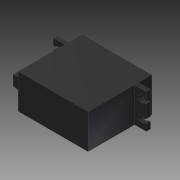
# Autodesk Inventor part: serwo HX12K
Saved by Autodesk Inventor 2013 (Build 170138000, 138)
## iProperties
Created: 2013-03-06
Part Number: serwo HX12K
Material: Generic
Document SubType Name: Modeling
Designer: Masta
Density: 1 g/cm^3
Author: Masta
Autodesk Inventor part; units mm, degrees
ref_plane "YZ Plane" through (0, 0, 0) normal (1, 0, 0) x (0, 1, 0)
ref_plane "XZ Plane" through (0, 0, 0) normal (0, 1, 0) x (-1, 0, 0)
ref_plane "XY Plane" through (0, 0, 0) normal (0, 0, 1) x (1, 0, 0)
sketch "Sketch1" plane through (0, 0, 0) normal (0, 1, 0) x (-1, 0, 0)
  line L0 (20.25, 10) -> (-20.25, 10)
  line L1 (-20.25, 10) -> (-20.25, -10)
  line L2 (-20.25, -10) -> (20.25, -10)
  line L3 (20.25, -10) -> (20.25, 10)
  line L4 (20.25, 10) -> (-20.25, -10) construction
  line L5 (-20.25, 10) -> (20.25, -10) construction
  line L6 (-27, 10) -> (-27, 6.25)
  line L7 (27, -10) -> (27, -6.25)
  line L8 (27, 10) -> (-27, -10) construction
  line L9 (-27, 10) -> (27, -10) construction
  line L10 (20.25, -10) -> (27, -10)
  line L11 (20.25, 10) -> (27, 10)
  line L12 (-20.25, 10) -> (-27, 10)
  line L13 (-20.25, -10) -> (-27, -10)
  line L14 (24.25, 5) -> (-24.25, 5) construction
  line L15 (-24.25, 5) -> (-24.25, -5) construction
  line L16 (-24.25, -5) -> (24.25, -5) construction
  line L17 (24.25, -5) -> (24.25, 5) construction
  line L18 (24.25, 5) -> (-24.25, -5) construction
  line L19 (-24.25, 5) -> (24.25, -5) construction
  circle A0 centre (-24.25, 5) radius 2
  line L20 (-27, 3.75) -> (-25.8112, 3.75)
  line L21 (-27, 6.25) -> (-25.8112, 6.25)
  line L22 (-20.25, 0) -> (20.25, 0) construction
  line L23 (0, 10) -> (0, -10) construction
  circle A1 centre (-24.25, -5) radius 2
  line L24 (-27, -3.75) -> (-25.8112, -3.75)
  line L25 (-27, -6.25) -> (-25.8112, -6.25)
  circle A2 centre (24.25, 5) radius 2
  line L26 (27, 3.75) -> (25.8112, 3.75)
  line L27 (27, 6.25) -> (25.8112, 6.25)
  line L28 (27, -6.25) -> (25.8112, -6.25)
  line L29 (27, -3.75) -> (25.8112, -3.75)
  circle A3 centre (24.25, -5) radius 2
  line L30 (-27, 3.75) -> (-27, -3.75)
  line L31 (-27, 6.25) -> (-27, 3.75)
  line L32 (-27, -6.25) -> (-27, -10)
  line L33 (-27, -3.75) -> (-27, -6.25)
  line L34 (27, -3.75) -> (27, 3.75)
  line L35 (27, -6.25) -> (27, -3.75)
  line L36 (27, 3.75) -> (27, 6.25)
  line L37 (27, 6.25) -> (27, 10)
  point P0 (0, 0)
  dimension "d0" = 40.5
  dimension "d1" = 20
  dimension "d2" = 54
  dimension "d3" = 48.5
  dimension "d4" = 10
  dimension "d12" = 2.5
  dimension "d13" = 4
  constraints: 76 end point, 32 parallel, 15 symmetric about line, 12 perpendicular, 10 midpoint, 8 point on circle, 4 centre point, 2 collinear, 2 horizontal, 1 coincident, 4 other
  measures "d0" distance of L2.end L1.end
  measures "d1" distance of L1.end L0.end
  measures "d2" distance of L7.start L8.end
  measures "d3" distance of L16.end L15.end
  measures "d4" distance of L15.end L14.end
  measures "d12" distance between parallel lines of L20 L21
  measures "d13" diameter of A0
extrude "Extrusion1" add sketch "Sketch1" along normal blind 10 and the other way blind 27 contours L3 L2 L1 L0
extrude "Extrusion2" add sketch "Sketch1" along normal blind 2.4 contours L11 L37 L27 A2 L26 L34 L29 A3 L28 L7 L10 L3 | L1 L13 L32 L25 A1 L24 L30 L20 A0 L21 L6 L12
sketch "Sketch2" plane through (0, 10, 0) normal (0, 1, 0) x (1, 0, 0)
  line L0 (-20.25, 10) -> (-20.25, -10) projected
  circle A0 centre (-10.25, 0) radius 6.5
  line L1 (-10.25, 0) -> (0, 0) construction
  dimension "d14" = 13
  dimension "d15" = 10
  constraints: 2 end point, 1 centre point, 1 perpendicular
  measures "d14" diameter of A0
  measures "d15" distance from line of L1.start L0
extrude "Extrusion3" add sketch "Sketch2" along normal blind 2
sketch "Sketch3" plane through (-10.25, 12, 0) normal (0, 1, 0) x (1, 0, 0)
  circle A0 centre (0, 0) radius 6.5 projected
  circle A1 centre (0, 0) radius 3
  point P0 (10.25, 0)
  dimension "d18" = 6
  constraints: 1 centre point, 1 coincident
  measures "d18" diameter of A1
extrude "Extrusion4" add sketch "Sketch3" along normal blind 4 contours A1
sketch "Sketch4" plane through (-20.25, -27, -10) normal (-1, 0, 0) x (0, 0, 1)
  line L0 (20, 27) -> (0, 27) projected
  line L1 (6.5, 3.5) -> (13.5, 3.5)
  line L2 (13.5, 3.5) -> (13.5, 8)
  line L3 (13.5, 8) -> (6.5, 8)
  line L4 (6.5, 8) -> (6.5, 3.5)
  line L5 (6.5, 3.5) -> (13.5, 8) construction
  line L6 (13.5, 3.5) -> (6.5, 8) construction
  line L7 (10, 27) -> (10, 5.75) construction
  dimension "d21" = 7
  dimension "d22" = 4.5
  dimension "d23" = 19
  constraints: 14 end point, 3 parallel, 2 midpoint, 1 horizontal, 1 perpendicular
  measures "d21" distance of L3.end L2.end
  measures "d22" distance of L2.end L1.end
  measures "d23" distance between parallel lines of L0 L3
extrude "Extrusion5" add sketch "Sketch4" along normal blind 7 draft -5
sketch "Sketch5" plane through (0, 0, 0) normal (0, 0, 1) x (1, 0, 0)
  line L0 (27, 2.4) -> (27, 0) projected
  line L1 (27, 0) -> (20.25, 0) projected
  line L2 (20.25, 0) -> (20.25, -27) projected
  line L3 (20.25, -27) -> (-20.25, -27) projected
  line L4 (-20.25, -27) -> (-20.25, -23.5) projected
  line L5 (-20.25, -23.5) -> (-27.25, -22.8876) projected
  line L6 (-27.25, -22.8876) -> (-27.25, -19.6124) projected
  line L7 (-27.25, -19.6124) -> (-20.25, -19) projected
  line L8 (-20.25, -19) -> (-20.25, 0) projected
  line L9 (-20.25, 0) -> (-27, 0) projected
  line L10 (-27, 0) -> (-27, 2.4) projected
  line L11 (-27, 2.4) -> (-20.25, 2.4) projected
  line L12 (-20.25, 2.4) -> (-20.25, 10) projected
  line L13 (-20.25, 10) -> (-16.75, 10) projected
  line L14 (-16.75, 10) -> (-16.75, 12) projected
  line L15 (-16.75, 12) -> (-13.25, 12) projected
  line L16 (-13.25, 12) -> (-13.25, 16) projected
  line L17 (-13.25, 16) -> (-7.25, 16) projected
  line L18 (-7.25, 16) -> (-7.25, 12) projected
  line L19 (-7.25, 12) -> (-3.75, 12) projected
  line L20 (-3.75, 12) -> (-3.75, 10) projected
  line L21 (-3.75, 10) -> (20.25, 10) projected
  line L22 (20.25, 10) -> (20.25, 2.4) projected
  line L23 (20.25, 2.4) -> (27, 2.4) projected
  line L24 (-27, 2.4) -> (-20.25, 3.5)
  line L25 (20.25, 3.5) -> (27, 2.4)
  point P0 (0, 0)
  dimension "d26" = 1.1
  constraints: 4 end point, 2 point on line, 1 equal length
  measures "d26" distance of L24.end L11.end
extrude "Extrusion6" add sketch "Sketch5" along normal mid plane 1.3 contours L23 L22 L25 | L24 L12 L11
sketch "Sketch6" plane through (0, 10, 0) normal (0, 1, 0) x (1, 0, 0)
  line L0 (12.3297, -7.1292) -> (12.3297, 6.9984) construction
  line L1 (12.3297, 6.9984) -> (15.9034, 6.9984) construction
  line L2 (15.9034, 6.9984) -> (15.9034, -7.1292) construction
  line L3 (15.9034, -7.1292) -> (12.3297, -7.1292) construction
  line L4 (15.9034, -4.2334) -> (15.9034, -4.6985)
  line L5 (15.9034, -4.6985) -> (14.1903, -4.6985)
  line L6 (14.1903, -4.6985) -> (14.1903, -6.3095)
  line L7 (14.1903, -6.3095) -> (15.9034, -6.3095)
  line L8 (15.9034, -6.3095) -> (15.9034, -6.7747)
  line L9 (15.9034, -6.7747) -> (12.4034, -6.7747)
  line L10 (12.4034, -6.7747) -> (12.4034, -6.3095)
  line L11 (12.4034, -6.3095) -> (13.7762, -6.3095)
  line L12 (13.7762, -6.3095) -> (13.7762, -4.6985)
  line L13 (13.7762, -4.6985) -> (12.4034, -4.6985)
  line L14 (12.4034, -4.6985) -> (12.4034, -4.2334)
  line L15 (12.4034, -4.2334) -> (15.9034, -4.2334)
  line L16 (15.9034, -1.1049) -> (15.9034, -1.6381)
  line L17 (15.9034, -1.6381) -> (14.508, -2.489)
  line L18 (14.508, -2.489) -> (15.9034, -3.3569)
  line L19 (15.9034, -3.3569) -> (15.9034, -3.859)
  line L20 (15.9034, -3.859) -> (14.1506, -2.7443)
  line L21 (14.1506, -2.7443) -> (12.4034, -3.8249)
  line L22 (12.4034, -3.8249) -> (12.4034, -3.2917)
  line L23 (12.4034, -3.2917) -> (13.7734, -2.4578)
  line L24 (13.7734, -2.4578) -> (12.4034, -1.6069)
  line L25 (12.4034, -1.6069) -> (12.4034, -1.1049)
  line L26 (12.4034, -1.1049) -> (14.1279, -2.1997)
  line L27 (14.1279, -2.1997) -> (15.9034, -1.1049)
  line L28 (15.9034, 1.1528) -> (15.9034, -0.5547)
  line L29 (15.9034, -0.5547) -> (15.5461, -0.5547)
  line L30 (15.5461, -0.5547) -> (15.5461, 0.0807)
  line L31 (15.5461, 0.0807) -> (13.2004, 0.0807)
  line L32 (13.2004, 0.0807) -> (13.2004, -0.5547)
  line L33 (13.2004, -0.5547) -> (12.8799, -0.5547)
  spline S0 degree 2 poles (12.8799, -0.5547) (12.8799, -0.1945) (12.6757, 0.1459) (12.3921, 0.1686) knots 0 0 0 1 2 2 2
  line L34 (12.3921, 0.1686) -> (12.3921, 0.5316)
  line L35 (12.3921, 0.5316) -> (15.5461, 0.5316)
  line L36 (15.5461, 0.5316) -> (15.5461, 1.1528)
  line L37 (15.5461, 1.1528) -> (15.9034, 1.1528)
  line L38 (15.9034, 3.955) -> (15.9034, 1.7966)
  line L39 (15.9034, 1.7966) -> (15.4071, 1.7966)
  spline S1 degree 2 poles (15.4071, 1.7966) (15.1887, 2.0292) (14.7831, 2.4433) (14.5647, 2.6418) knots 0 0 0 1 2 2 2
  spline S2 degree 2 poles (14.5647, 2.6418) (14.1251, 3.0418) (13.5975, 3.3339) (13.3167, 3.3339) knots 0 0 0 1 2 2 2
  spline S3 degree 2 poles (13.3167, 3.3339) (13.1692, 3.3339) (12.948, 3.2431) (12.8771, 3.1609) knots 0 0 0 1 2 2 2
  spline S4 degree 2 poles (12.8771, 3.1609) (12.8062, 3.0786) (12.7353, 2.8631) (12.7353, 2.7326) knots 0 0 0 1 2 2 2
  spline S5 degree 2 poles (12.7353, 2.7326) (12.7353, 2.6078) (12.7977, 2.3525) (12.8459, 2.2362) knots 0 0 0 1 2 2 2
  spline S6 degree 2 poles (12.8459, 2.2362) (12.8856, 2.137) (12.9991, 1.9526) (13.0388, 1.8959) knots 0 0 0 1 2 2 2
  line L40 (13.0388, 1.8959) -> (13.0388, 1.8704)
  line L41 (13.0388, 1.8704) -> (12.5396, 1.8704)
  spline S7 degree 2 poles (12.5396, 1.8704) (12.4687, 2.015) (12.3297, 2.5341) (12.3297, 2.7666) knots 0 0 0 1 2 2 2
  spline S8 degree 2 poles (12.3297, 2.7666) (12.3297, 3.2573) (12.8487, 3.8104) (13.2912, 3.8104) knots 0 0 0 1 2 2 2
  spline S9 degree 2 poles (13.2912, 3.8104) (13.4982, 3.8104) (13.8443, 3.714) (13.9918, 3.6289) knots 0 0 0 1 2 2 2
  spline S10 degree 2 poles (13.9918, 3.6289) (14.1449, 3.5438) (14.4456, 3.297) (14.5902, 3.1609) knots 0 0 0 1 2 2 2
  spline S11 degree 2 poles (14.5902, 3.1609) (14.8313, 2.9396) (15.3475, 2.3979) (15.4978, 2.2362) knots 0 0 0 1 2 2 2
  line L42 (15.4978, 2.2362) -> (15.4978, 3.955)
  line L43 (15.4978, 3.955) -> (15.9034, 3.955)
  line L44 (15.9034, 7.075) -> (15.9034, 6.4708)
  line L45 (15.9034, 6.4708) -> (14.2754, 5.1917)
  line L46 (14.2754, 5.1917) -> (14.5051, 4.9875)
  line L47 (14.5051, 4.9875) -> (15.9034, 4.9875)
  line L48 (15.9034, 4.9875) -> (15.9034, 4.5223)
  line L49 (15.9034, 4.5223) -> (12.4034, 4.5223)
  line L50 (12.4034, 4.5223) -> (12.4034, 4.9875)
  line L51 (12.4034, 4.9875) -> (14.0116, 4.9875)
  line L52 (14.0116, 4.9875) -> (12.4034, 6.4226)
  line L53 (12.4034, 6.4226) -> (12.4034, 6.9899)
  line L54 (12.4034, 6.9899) -> (13.9662, 5.5405)
  line L55 (13.9662, 5.5405) -> (15.9034, 7.075)
  point P0 (0, 0)
  constraints: 2 other
emboss "Emboss1" sketch "Sketch6" operation cut depth 0.1 direction (0, -1, 0)
hole "Hole1" at (-10.25, 16, 0) direction (0, -1, 0) diameter 2.459 depth 8 tip angle 118 thread size "M3x0.5" class "6H" standard "ISO Metric profile"
body "Solid1"
